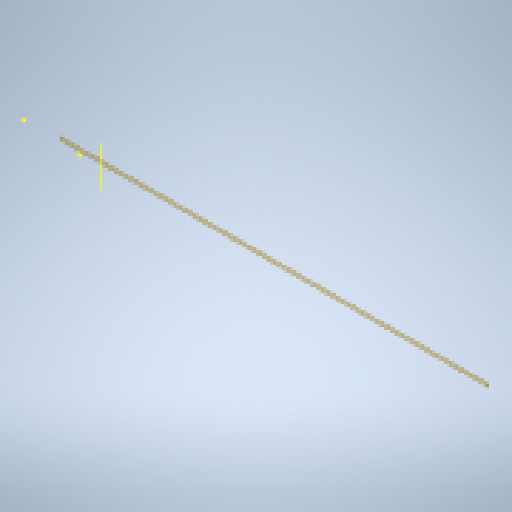
# Autodesk Inventor part: GantryAxisHolder
Saved by Autodesk Inventor 2023 (Build 270158000, 158)
## iProperties
Created: 2023-09-08
Part Number: GantryAxisHolder
Material: Generic
Document SubType Name: Modeling
Designer: Felix
Density: 1 g/cm^3
Appearance: Default
Author: Felix
Autodesk Inventor part; units mm, degrees
ref_plane "YZ Plane" through (0, 0, 0) normal (1, 0, 0) x (0, 1, 0)
ref_plane "XZ Plane" through (0, 0, 0) normal (0, 1, 0) x (-1, 0, 0)
ref_plane "XY Plane" through (0, 0, 0) normal (0, 0, 1) x (1, 0, 0)
ref_plane "Work Plane1" through (88.049, 6.8107, 7.4208) normal (0, 0, 1) x (0, -1, 0)
sketch "Sketch1" plane through (88.049, 6.8107, 7.4208) normal (0, 0, 1) x (0, -1, 0)
  circle A0 centre (8.5, 0) radius 2.55 construction
  line L0 (38.25, 32.75) -> (-21.25, 32.75) projected
  circle A1 centre (8.5, -19.85) radius 4 construction
  line L1 (8.5, -19.85) -> (8.5, 20) construction
  line L2 (16, -19.85) -> (16, 20)
  line L3 (1, 20) -> (1, -19.85)
  arc A2 (1, -19.85) -> (16, -19.85) centre (8.5, -19.85) ccw
  arc A3 (16, 20) -> (1, 20) centre (8.5, 20) ccw
  point P0 (6.8107, -88.049)
  point P1 (8.5, 0.075)
  dimension "d0" = 15
  dimension "d20" = 20
  constraints: 8 end point, 4 point on circle, 4 tangent, 2 centre point, 1 midpoint, 1 parallel, 1 vertical
  measures "d0" diameter of A3
  measures "d20" distance of L1.end A0.centre
extrude "Extrusion1" add sketch "Sketch1" along normal blind 5
sketch "Sketch2" plane through (88.049, 6.8107, 12.4208) normal (0, 0, 1) x (1, 0, 0)
  circle A0 centre (-19.85, -8.5) radius 4 construction
  circle A1 centre (0, -8.5) radius 2.55 construction
  line L0 (0, -8.5) -> (22.0742, -8.5) construction
  point P0 (-88.049, -6.8107)
  point P1 (10, -8.5)
  point P2 (20, -8.5)
  dimension "d4" = 10
  dimension "d5" = 10
  constraints: 2 end point, 2 point on line, 1 coincident, 1 horizontal
  measures "d4" distance of point (10, -8.5) L0.start
  measures "d5" distance of point (20, -8.5) point (10, -8.5)
hole "Hole1" at (98.049, -1.6893, 12.4208) at (108.049, -1.6893, 12.4208) direction (0, 0, -1) diameter 4.5 depth 6 clearance for "Countersunk Flat Head Screw DIN EN ISO 2009" size "M4" standard "DIN"
sketch "Sketch3" plane through (88.049, 6.8107, 12.4208) normal (0, 0, 1) x (1, 0, 0)
  point P0 (-88.049, -6.8107)
  point P1 (-19.85, -8.5)
hole "Hole2" at (68.199, -1.6893, 12.4208) direction (0, 0, -1) diameter 9 depth 6 clearance for "Slotted Cheese Head Screw DIN 84" size "M8" standard "DIN"
body "Solid1"
